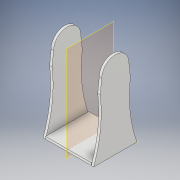
# Autodesk Inventor part: MAN_BASIS_PRIMARY_STRUCTURE
Saved by Autodesk Inventor 2019 (Build 230136000, 136)
## iProperties
Created: 2021-03-07
Part Number: MAN_BASIS_PRIMARY_STRUCTURE
Material: ABS Plastic
Document SubType Name: Modeling
Designer: DOMEK
Density: 1.06 g/cm^3
Appearance: Smooth - White
Author: DOMEK
Autodesk Inventor part; units mm, degrees
ref_plane "YZ Plane" through (0, 0, 0) normal (1, 0, 0) x (0, 1, 0)
ref_plane "XZ Plane" through (0, 0, 0) normal (0, 1, 0) x (-1, 0, 0)
ref_plane "XY Plane" through (0, 0, 0) normal (0, 0, 1) x (1, 0, 0)
sketch "Sketch7" plane through (0, 0, 0) normal (0, 1, 0) x (-1, 0, 0)
  line L0 (0, 0) -> (41, 0)
  line L1 (41, 0) -> (41, 35)
  line L2 (41, 35) -> (0, 35)
  line L3 (0, 35) -> (0, 0)
  dimension "d20" = 41
  dimension "d21" = 35
  constraints: 8 end point, 2 parallel, 1 horizontal, 1 perpendicular
  measures "d20" distance of L2.end L1.end
  measures "d21" distance of L1.end L0.end
extrude "Extrusion6" add sketch "Sketch7" along normal blind 70
shell "Shell1" thickness 2 removed faces 3 at (-13.6667, 70, 23.3333) at (-27.3333, 23.3333, 35) at (-13.6667, 23.3333, 0)
sketch "Sketch8" plane through (0, 0, 35) normal (1, 0, 0) x (0, 0, -1)
  point P0 (35, 0)
sketch "Sketch9" plane through (0, 0, 35) normal (1, 0, 0) x (0, 0, -1)
  line L0 (0, 70) -> (35, 70) projected
  line L1 (17.5, 70) -> (17.5, 0)
  arc A0 (35, 70) -> (35, 0) centre (132.4173, 35) ccw
  arc A1 (0, 0) -> (0, 70) centre (-97.4173, 35) ccw
  line L2 (35, 70) -> (35, 2) projected
  line L3 (35, 0) -> (35, 70)
  line L4 (35, 0) -> (0, 0) projected
  line L5 (0, 0) -> (0, 70) projected
  line L6 (0, 0) -> (0, 70)
  constraints: 6 end point, 4 point on circle, 2 centre point, 2 collinear, 2 symmetric about line, 1 midpoint, 1 vertical, 1 other
extrude "Extrusion7" cut sketch "Sketch9" against normal blind 2 contours A1 L5 | L2 L3 A0
ref_plane "Work Plane6" through (-20.5, 0, 35) normal (1, 0, 0) x (0, 0, -1)
mirror "Mirror3" about plane through (-20.5, 0, 35) normal (1, 0, 0) of "Extrusion7"
sketch "Sketch10" plane through (0, 0, 35) normal (1, 0, 0) x (0, 0, -1)
  line L0 (0, 70) -> (35, 70) projected
  line L1 (17.5, 70) -> (17.5, 59)
  circle A0 centre (17.5, 59) radius 11
  line L2 (28.5, 59) -> (29.7229, 48)
  arc A1 (35, 70) -> (34.3045, 2) centre (132.4173, 35) ccw projected
  line L3 (6.5, 59) -> (5.2771, 48)
  arc A2 (0.6955, 2) -> (0, 70) centre (-97.4173, 35) ccw projected
  point P0 (35, 0)
  dimension "d30" = 11
  dimension "d31" = 22
  constraints: 6 end point, 4 point on circle, 1 centre point, 1 coincident, 1 midpoint, 1 vertical
  measures "d30" distance of L1.start L1.end
  measures "d31" diameter of A0
extrude "Extrusion8" cut sketch "Sketch10" against normal blind 2 contours L0 A0 L3 A2 | L0 A1 L2 A0
mirror "Mirror4" about plane through (-20.5, 0, 35) normal (1, 0, 0) of "Extrusion8"
body "Solid2"
